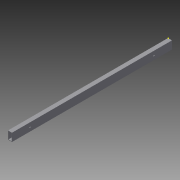
# Autodesk Inventor part: 40in 2x1 boxbeam
Saved by Autodesk Inventor 2015 (Build 190159000, 159)
## iProperties
Created: 2015-01-11
Part Number: 40in 2x1 boxbeam
Material: Generic
Document SubType Name: Modeling
Designer: chapale16
Density: 1 g/cm^3
Appearance: Default
Author: chapale16
Autodesk Inventor part; units mm, degrees
ref_plane "YZ Plane" through (0, 0, 0) normal (1, 0, 0) x (0, 1, 0)
ref_plane "XZ Plane" through (0, 0, 0) normal (0, 1, 0) x (-1, 0, 0)
ref_plane "XY Plane" through (0, 0, 0) normal (0, 0, 1) x (1, 0, 0)
sketch "Sketch1" plane through (0, 0, 0) normal (0, 0, 1) x (1, 0, 0)
  line L0 (-2.7678, 3.3517) -> (22.6322, 3.3517)
  line L1 (22.6322, 3.3517) -> (22.6322, -47.4483)
  line L2 (22.6322, -47.4483) -> (-2.7678, -47.4483)
  line L3 (-2.7678, -47.4483) -> (-2.7678, 3.3517)
  line L4 (19.5061, 0.2256) -> (0.3583, 0.2256)
  line L5 (0.3583, 0.2256) -> (0.3583, -44.3222)
  line L6 (0.3583, -44.3222) -> (19.5061, -44.3222)
  line L7 (19.5061, -44.3222) -> (19.5061, 0.2256)
  point P0 (0, 0)
  dimension "d0" = 25.4
  dimension "d1" = 50.8
  constraints: 16 end point, 4 parallel, 2 perpendicular, 1 horizontal, 3 other
  measures "d0" distance of L1.end L2.end
  measures "d1" distance of L0.end L1.end
extrude "Extrusion1" add sketch "Sketch1" along normal blind 1016
sketch "Sketch2" plane through (-2.7678, 3.3517, 0) normal (0, 1, 0) x (1, 0, 0)
  point P0 (2.7678, 0)
sketch "Sketch3" plane through (22.6322, -47.4483, 0) normal (1, 0, 0) x (0, 0, -1)
  line L0 (0, 0) -> (-1016, 0) projected
  line L1 (0, 50.8) -> (-114.3, 50.8)
  line L2 (-114.3, 50.8) -> (-114.3, 0)
  line L3 (-114.3, 0) -> (0, 0)
  line L4 (0, 0) -> (0, 50.8)
  line L5 (-1016, 50.8) -> (-901.7, 50.8)
  line L6 (-901.7, 50.8) -> (-901.7, 0)
  line L7 (-901.7, 0) -> (-1016, 0)
  line L8 (-1016, 0) -> (-1016, 50.8)
  point P0 (0, 47.4483)
  point P1 (-114.3, 25.4)
  point P2 (-901.7, 25.4)
  dimension "d4" = 114.3
  dimension "d5" = 114.3
  constraints: 16 end point, 4 parallel, 2 horizontal, 2 midpoint, 2 perpendicular, 2 point on line
  measures "d4" distance of L3.end L2.end
  measures "d5" distance of L6.end L7.end
hole "Hole1" at (22.6322, -22.0483, 901.7) at (22.6322, -22.0483, 114.3) direction (-1, 0, 0) diameter 9.525 end through all
body "Solid1"
